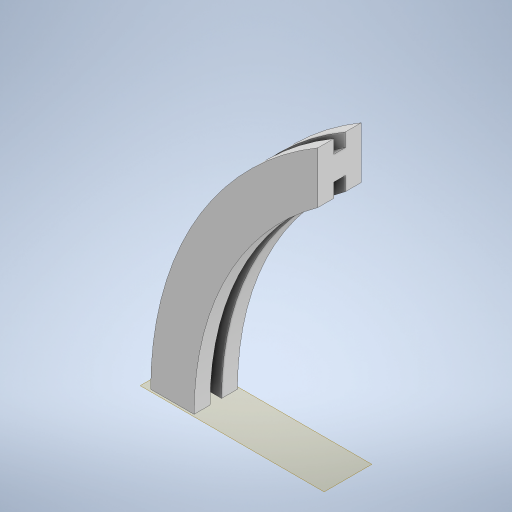
# Autodesk Inventor part: LightRail01
Saved by Autodesk Inventor 2023 (Build 270158000, 158)
## iProperties
Created: 2023-04-11
Part Number: LightRail01
Material: Generic
Document SubType Name: Modeling
Designer: ringl
Density: 1 g/cm^3
Appearance: Default
Author: ringl
Autodesk Inventor part; units mm, degrees
ref_plane "YZ Plane" through (0, 0, 0) normal (1, 0, 0) x (0, 1, 0)
ref_plane "XY Plane" through (0, 0, 0) normal (0, 0, 1) x (1, 0, 0)
sketch "Sketch1" plane through (0, 0, 0) normal (0, 0, 1) x (1, 0, 0)
  arc A0 (440, 0) -> (0, 0) centre (220, 0) ccw
  dimension "d1" = 440
  dimension "d17" = 220
  constraints: 2 point on circle, 1 centre point, 1 horizontal alignment
  measures "d1" distance of A0.end A0.start
  measures "d17" radius of A0
sketch "Sketch2" plane through (0, 0, 0) normal (0, 1, 0) x (-1, 0, 0)
  line L0 (15, 15) -> (-15, 15)
  line L1 (-15, -15) -> (15, -15)
  line L2 (15, 4) -> (7, 4)
  line L3 (7, 4) -> (7, -4)
  line L4 (7, -4) -> (15, -4)
  line L5 (-15, 4) -> (-7, 4)
  line L6 (-7, 4) -> (-7, -4)
  line L7 (-7, -4) -> (-15, -4)
  line L8 (15, -15) -> (15, -4)
  line L9 (15, 4) -> (15, 15)
  line L10 (-15, 15) -> (-15, 4)
  line L11 (-15, -4) -> (-15, -15)
  point P0 (0, 0)
  dimension "d18" = 8
  dimension "d19" = 8
  dimension "d21" = 14
  dimension "d22" = 30
  dimension "d23" = 15
  dimension "d24" = 4
  dimension "d25" = 7
  constraints: 24 end point, 7 parallel, 4 perpendicular, 3 equal length, 3 horizontal, 2 point on line
  measures "d18" distance of L5.end L6.end
  measures "d19" distance of L5.start L5.end
  measures "d21" distance between parallel lines of L3 L6
  measures "d22" distance between parallel lines of L1 L0
  measures "d23" distance from line of L1 point (0, 0)
  measures "d24" distance from line of point (0, 0) L5
  measures "d25" distance from line of L6 point (0, 0)
sweep "Sweep1" add profiles "Sketch2" path "Sketch1"
sketch "Sketch3" plane through (-15, 0, 15) normal (0, 0, 1) x (1, 0, 0)
  line L0 (472.3789, 0) -> (115.6515, 0)
  line L1 (115.6515, 0) -> (115.6515, 304.2951)
  line L2 (115.6515, 304.2951) -> (472.3789, 304.2951)
  line L3 (472.3789, 304.2951) -> (472.3789, 0)
  line L4 (0, 0) -> (30, 0) projected
  point P0 (15, 0)
  point P1 (15, 0)
  point P2 (15, 0)
  dimension "d28" = 356.7274
  dimension "d29" = 304.2951
  dimension "d30" = 100.6515
  dimension "d31" = 0
  constraints: 8 end point, 2 midpoint, 2 parallel, 1 horizontal, 1 perpendicular
  measures "d28" distance of L1.end L2.end
  measures "d29" distance of L0.end L1.end
  measures "d30" distance of point (15, 0) L0.end
  measures "d31" vertical distance of point (15, 0) L0.end
extrude "Extrusion1" cut sketch "Sketch3" against normal through all
body "Solid1"
